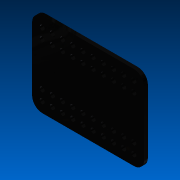
# Autodesk Inventor part: ROV-Bottom Panel
Saved by Autodesk Inventor 2013 (Build 170138000, 138)
## iProperties
Created: 2014-11-06
Part Number: ROV-Bottom Panel
Material: Acetal Resin, Black
Document SubType Name: Modeling
Designer: Jeramy
Density: 1 g/cm^3
Author: Jeramy
Autodesk Inventor part; units mm, degrees
ref_plane "YZ Plane" through (0, 0, 0) normal (1, 0, 0) x (0, 1, 0)
ref_plane "XZ Plane" through (0, 0, 0) normal (0, 1, 0) x (-1, 0, 0)
ref_plane "XY Plane" through (0, 0, 0) normal (0, 0, 1) x (1, 0, 0)
sketch "Sketch1" plane through (0, 0, 0) normal (0, 0, 1) x (1, 0, 0)
  line L0 (0, 0) -> (558.8, 0)
  line L1 (558.8, 0) -> (558.8, 419.1)
  line L2 (558.8, 419.1) -> (0, 419.1)
  line L3 (0, 419.1) -> (0, 0)
  dimension "d0" = 558.8
  dimension "d1" = 419.1
  constraints: 8 end point, 2 parallel, 1 horizontal, 1 perpendicular
  measures "d0" distance of L2.end L1.end
  measures "d1" distance of L1.end L0.end
extrude "Extrusion1" add sketch "Sketch1" along normal blind 19.05
fillet "Fillet1" radius 50.8 1 edges at (558.8, 419.1, 9.525)
fillet "Fillet2" radius 50.8 1 edges at (558.8, 0, 9.525)
fillet "Fillet3" radius 50.8 1 edges at (0, 419.1, 9.525)
fillet "Fillet4" radius 50.8 1 edges at (0, 0, 9.525)
sketch "Sketch2" plane through (0, 0, 19.05) normal (0, 0, 1) x (1, 0, 0)
  arc A0 (558.8, 368.3) -> (508, 419.1) centre (508, 368.3) ccw projected
  line L0 (0, 368.3) -> (0, 50.8) projected
  circle A1 centre (50.8, 368.3) radius 12.7
  line L1 (50.8, 368.3) -> (101.6, 368.3)
  line L2 (101.6, 368.3) -> (101.6, 317.5)
  line L3 (50.8, 368.3) -> (50.8, 317.5)
  line L4 (101.6, 368.3) -> (152.4, 368.3)
  line L5 (152.4, 368.3) -> (203.2, 368.3)
  line L6 (203.2, 368.3) -> (254, 368.3)
  line L7 (254, 368.3) -> (304.8, 368.3)
  line L8 (304.8, 368.3) -> (355.6, 368.3)
  line L9 (355.6, 368.3) -> (406.4, 368.3)
  line L10 (406.4, 368.3) -> (457.2, 368.3)
  line L11 (457.2, 368.3) -> (508, 368.3)
  line L12 (508, 368.3) -> (508, 317.5)
  line L13 (457.2, 368.3) -> (457.2, 317.5)
  line L14 (406.4, 368.3) -> (406.4, 317.5)
  line L15 (355.6, 368.3) -> (355.6, 317.5)
  line L16 (304.8, 368.3) -> (304.8, 317.5)
  line L17 (254, 368.3) -> (254, 317.5)
  line L18 (203.2, 368.3) -> (203.2, 317.5)
  line L19 (152.4, 368.3) -> (152.4, 317.5)
  circle A2 centre (101.6, 368.3) radius 12.7
  circle A3 centre (152.4, 368.3) radius 12.7
  circle A4 centre (203.2, 368.3) radius 12.7
  circle A5 centre (254, 368.3) radius 12.7
  circle A6 centre (304.8, 368.3) radius 12.7
  circle A7 centre (355.6, 368.3) radius 12.7
  circle A8 centre (406.4, 368.3) radius 12.7
  circle A9 centre (457.2, 368.3) radius 12.7
  circle A10 centre (508, 368.3) radius 12.7
  circle A11 centre (508, 317.5) radius 12.7
  circle A12 centre (457.2, 317.5) radius 12.7
  circle A13 centre (406.4, 317.5) radius 12.7
  circle A14 centre (355.6, 317.5) radius 12.7
  circle A15 centre (304.8, 317.5) radius 12.7
  circle A16 centre (254, 317.5) radius 12.7
  circle A17 centre (203.2, 317.5) radius 12.7
  circle A18 centre (152.4, 317.5) radius 12.7
  circle A19 centre (101.6, 317.5) radius 12.7
  circle A20 centre (50.8, 317.5) radius 12.7
  circle A21 centre (50.8, 101.6) radius 12.7
  line L20 (50.8, 101.6) -> (101.6, 101.6)
  line L21 (101.6, 101.6) -> (101.6, 50.8)
  line L22 (50.8, 101.6) -> (50.8, 50.8)
  line L23 (101.6, 101.6) -> (152.4, 101.6)
  line L24 (152.4, 101.6) -> (203.2, 101.6)
  line L25 (203.2, 101.6) -> (254, 101.6)
  line L26 (254, 101.6) -> (304.8, 101.6)
  line L27 (304.8, 101.6) -> (355.6, 101.6)
  line L28 (355.6, 101.6) -> (406.4, 101.6)
  line L29 (406.4, 101.6) -> (457.2, 101.6)
  line L30 (457.2, 101.6) -> (508, 101.6)
  line L31 (508, 101.6) -> (508, 50.8)
  line L32 (457.2, 101.6) -> (457.2, 50.8)
  line L33 (406.4, 101.6) -> (406.4, 50.8)
  line L34 (355.6, 101.6) -> (355.6, 50.8)
  line L35 (304.8, 101.6) -> (304.8, 50.8)
  line L36 (254, 101.6) -> (254, 50.8)
  line L37 (203.2, 101.6) -> (203.2, 50.8)
  line L38 (152.4, 101.6) -> (152.4, 50.8)
  circle A22 centre (101.6, 101.6) radius 12.7
  circle A23 centre (152.4, 101.6) radius 12.7
  circle A24 centre (203.2, 101.6) radius 12.7
  circle A25 centre (254, 101.6) radius 12.7
  circle A26 centre (304.8, 101.6) radius 12.7
  circle A27 centre (355.6, 101.6) radius 12.7
  circle A28 centre (406.4, 101.6) radius 12.7
  circle A29 centre (457.2, 101.6) radius 12.7
  circle A30 centre (508, 101.6) radius 12.7
  circle A31 centre (508, 50.8) radius 12.7
  circle A32 centre (457.2, 50.8) radius 12.7
  circle A33 centre (406.4, 50.8) radius 12.7
  circle A34 centre (355.6, 50.8) radius 12.7
  circle A35 centre (304.8, 50.8) radius 12.7
  circle A36 centre (254, 50.8) radius 12.7
  circle A37 centre (203.2, 50.8) radius 12.7
  circle A38 centre (152.4, 50.8) radius 12.7
  circle A39 centre (101.6, 50.8) radius 12.7
  circle A40 centre (50.8, 50.8) radius 12.7
  point P0 (0, 0)
  dimension "d8" = 25.4
  dimension "d9" = 50.8
  dimension "d10" = 50.8
  dimension "d11" = 50.8
  dimension "d12" = 50.8
  dimension "d13" = 50.8
  dimension "d14" = 50.8
  dimension "d15" = 50.8
  dimension "d16" = 50.8
  dimension "d17" = 50.8
  dimension "d18" = 50.8
  dimension "d19" = 50.8
  dimension "d20" = 50.8
  dimension "d21" = 50.8
  dimension "d22" = 50.8
  dimension "d23" = 50.8
  dimension "d24" = 50.8
  dimension "d25" = 50.8
  dimension "d26" = 50.8
  dimension "d27" = 50.8
  dimension "d28" = 25.4
  dimension "d29" = 25.4
  dimension "d30" = 25.4
  dimension "d31" = 25.4
  dimension "d32" = 25.4
  dimension "d33" = 25.4
  dimension "d34" = 25.4
  dimension "d35" = 25.4
  dimension "d36" = 25.4
  dimension "d37" = 25.4
  dimension "d38" = 25.4
  dimension "d39" = 25.4
  dimension "d40" = 25.4
  dimension "d41" = 25.4
  dimension "d42" = 25.4
  dimension "d43" = 25.4
  dimension "d44" = 25.4
  dimension "d45" = 25.4
  dimension "d46" = 25.4
  dimension "d47" = 25.4
  dimension "d48" = 50.8
  dimension "d49" = 50.8
  dimension "d50" = 50.8
  dimension "d51" = 50.8
  dimension "d52" = 50.8
  dimension "d53" = 50.8
  dimension "d54" = 50.8
  dimension "d55" = 50.8
  dimension "d56" = 50.8
  dimension "d57" = 50.8
  dimension "d58" = 50.8
  dimension "d59" = 50.8
  dimension "d60" = 50.8
  dimension "d61" = 50.8
  dimension "d62" = 50.8
  dimension "d63" = 50.8
  dimension "d64" = 50.8
  dimension "d65" = 50.8
  dimension "d66" = 50.8
  dimension "d67" = 25.4
  dimension "d68" = 25.4
  dimension "d69" = 25.4
  dimension "d70" = 25.4
  dimension "d71" = 25.4
  constraints: 76 end point, 40 centre point, 30 equal length, 7 perpendicular
  measures "d8" diameter of A1
  measures "d9" distance of L1.start L1.end
  measures "d10" distance of L1.end L2.end
  measures "d11" distance of L1.start L3.end
  measures "d12" distance of L1.end L4.end
  measures "d13" distance of L4.end L5.end
  measures "d14" distance of L5.end L6.end
  measures "d15" distance of L6.end L7.end
  measures "d16" distance of L7.end L8.end
  measures "d17" distance of L8.end L9.end
  measures "d18" distance of L9.end L10.end
  measures "d19" distance of L10.end L11.end
  measures "d20" distance of L11.end L12.end
  measures "d21" distance of L10.end L13.end
  measures "d22" distance of L9.end L14.end
  measures "d23" distance of L8.end L15.end
  measures "d24" distance of L7.end L16.end
  measures "d25" distance of L6.end L17.end
  measures "d26" distance of L5.end L18.end
  measures "d27" distance of L4.end L19.end
  measures "d28" diameter of A2
  measures "d29" diameter of A3
  measures "d30" diameter of A4
  measures "d31" diameter of A5
  measures "d32" diameter of A6
  measures "d33" diameter of A7
  measures "d34" diameter of A8
  measures "d35" diameter of A9
  measures "d36" diameter of A10
  measures "d37" diameter of A11
  measures "d38" diameter of A12
  measures "d39" diameter of A13
  measures "d40" diameter of A14
  measures "d41" diameter of A15
  measures "d42" diameter of A16
  measures "d43" diameter of A17
  measures "d44" diameter of A18
  measures "d45" diameter of A19
  measures "d46" diameter of A20
  measures "d47" diameter of A21
  measures "d48" distance of L20.start L20.end
  measures "d49" distance of L20.end L21.end
  measures "d50" distance of L20.start L22.end
  measures "d51" distance of L20.end L38.start
  measures "d52" distance of L38.start L24.end
  measures "d53" distance of L24.end L26.start
  measures "d54" distance of L26.start L26.end
  measures "d55" distance of L26.end L28.start
  measures "d56" distance of L28.start L28.end
  measures "d57" distance of L28.end L29.end
  measures "d58" distance of L29.end L31.start
  measures "d59" distance of L31.start L31.end
  measures "d60" distance of L29.end L32.end
  measures "d61" distance of L28.end L33.end
  measures "d62" distance of L28.start L34.end
  measures "d63" distance of L26.end L35.end
  measures "d64" distance of L26.start L36.end
  measures "d65" distance of L24.end L37.end
  measures "d66" distance of L38.start L38.end
  measures "d67" diameter of A22
  measures "d68" diameter of A23
  measures "d69" diameter of A24
  measures "d70" diameter of A25
  measures "d71" diameter of A26
extrude "Extrusion2" cut sketch "Sketch2" against normal blind 19.05
body "Solid1"
